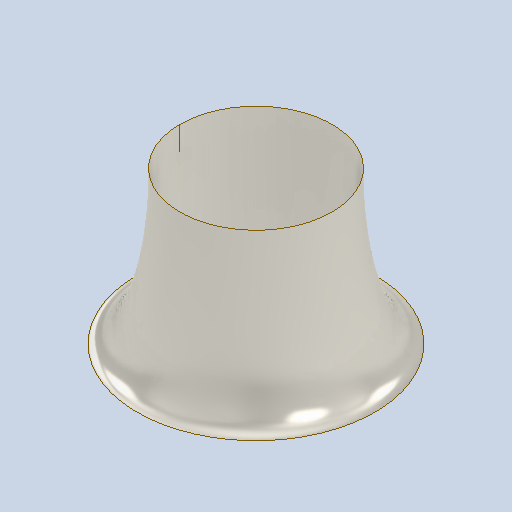
# Autodesk Inventor part: TorsOsc-202511-rod-coupling-solder
Saved by Autodesk Inventor 2026 (Build 300175050, 175E)
## iProperties
Created: 2023-08-21
Part Number: TorsOsc-202511-rod-coupling-solder
Material: Titanium
Document SubType Name: Modeling
Designer: schanen
Density: 4.51 g/cm^3
Appearance: Titanium
Author: schanen
Autodesk Inventor part; units mm, degrees
ref_plane "YZ Plane" through (0, 0, 0) normal (1, 0, 0) x (0, 1, 0)
ref_plane "XZ Plane" through (0, 0, 0) normal (0, 1, 0) x (-1, 0, 0)
ref_plane "XY Plane" through (0, 0, 0) normal (0, 0, 1) x (1, 0, 0)
sketch "Sketch1" plane through (0, 0, 0) normal (0, 0, 1) x (1, 0, 0)
  line L0 (-0.4, 0) -> (-0.4, 0.8)
  line L1 (-0.4, 0) -> (-0.625, 0)
  ellipse E0 centre (-0.625, 0.8) end of major axis (-0.625, 0) minor radius 0.225
  line L2 (0, -0.32) -> (0, 1.92) projected
  point P0 (0, 0)
  dimension "d0" = 0.625
  dimension "d1" = 0.4
  dimension "d2" = 0.8
  constraints: 4 end point, 2 horizontal alignment, 1 horizontal, 1 vertical, 1 vertical alignment, 4 other
  measures "d0" distance of point (0, 0) L1.end
  measures "d1" distance from line of point (0, 0) L0
  measures "d2" distance of L0.start L0.end
revolve "Revolution1" add sketch "Sketch1" angle 360 about axis through (0, -10, 0) along (0, 1, 0) contours L1 E0 L0
body "Solid1"
